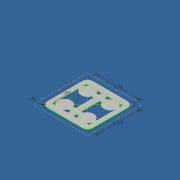
# Autodesk Inventor part: PCB Dome Array Tape
Saved by Autodesk Inventor 2016 (Build 200138000, 138)
## iProperties
Created: 2016-02-25
Part Number: PCB Dome Array Tape
Material: Generic
Document SubType Name: Modeling
Designer: Sam Clay
Density: 1 g/cm^3
Appearance: Default
Author: Sam Clay
Autodesk Inventor part; units mm, degrees
ref_plane "YZ Plane" through (0, 0, 0) normal (1, 0, 0) x (0, 1, 0)
ref_plane "XZ Plane" through (0, 0, 0) normal (0, 1, 0) x (-1, 0, 0)
ref_plane "XY Plane" through (0, 0, 0) normal (0, 0, 1) x (1, 0, 0)
sketch "Sketch1" plane through (0, 0, 0) normal (0, 1, 0) x (-1, 0, 0)
  line L0 (-15.24, 11.7348) -> (-15.24, -11.7348)
  line L1 (-11.7348, -15.24) -> (11.7348, -15.24)
  line L2 (15.24, -11.7348) -> (15.24, 11.7348)
  line L3 (11.7348, 15.24) -> (-11.7348, 15.24)
  line L4 (-15.24, 15.24) -> (15.24, -15.24) construction
  line L5 (-15.24, -15.24) -> (15.24, 15.24) construction
  arc A0 (15.24, 11.7348) -> (11.7348, 15.24) centre (11.7348, 11.7348) ccw
  arc A1 (11.7348, -15.24) -> (15.24, -11.7348) centre (11.7348, -11.7348) ccw
  arc A2 (-15.24, -11.7348) -> (-11.7348, -15.24) centre (-11.7348, -11.7348) ccw
  arc A3 (-11.7348, 15.24) -> (-15.24, 11.7348) centre (-11.7348, 11.7348) ccw
  line L6 (-18.4479, 18.3502) -> (18.4026, 18.3502) construction
  line L7 (18.4026, 18.3502) -> (18.4026, -18.5003) construction
  line L8 (18.4026, -18.5003) -> (-18.4479, -18.5003) construction
  line L9 (-18.4479, -18.5003) -> (-18.4479, 18.3502) construction
  line L10 (12.7, 11.7348) -> (12.7, 9.1616)
  arc A4 (11.7348, -12.7) -> (12.7, -11.7348) centre (11.7348, -11.7348) ccw
  line L11 (11.7348, -12.7) -> (-11.7348, -12.7)
  arc A5 (-12.7, -11.7348) -> (-11.7348, -12.7) centre (-11.7348, -11.7348) ccw
  line L12 (-12.7, -11.7348) -> (-12.7, -9.2677)
  arc A6 (-11.7348, 12.7) -> (-12.7, 11.7348) centre (-11.7348, 11.7348) ccw
  line L13 (-11.7348, 12.7) -> (11.7348, 12.7)
  arc A7 (12.7, 11.7348) -> (11.7348, 12.7) centre (11.7348, 11.7348) ccw
  line L14 (12.7, 9.1616) -> (1.5905, 9.1616)
  line L15 (-12.7, 9.1616) -> (-12.7, 11.7348)
  line L16 (-12.7, 11.7348) -> (-1.7389, 11.7348)
  line L17 (12.7, 11.7348) -> (12.7, 9.1616)
  line L18 (12.7, -9.2677) -> (1.5905, -9.2677)
  line L19 (-12.7, -9.2677) -> (-12.7, -11.7348)
  line L20 (-12.7, -11.7348) -> (-1.7389, -11.7348)
  line L21 (12.7, -11.7348) -> (12.7, -9.2677)
  line L22 (-12.7, 9.1616) -> (-12.7, 11.7348)
  line L23 (12.7, 6.4035) -> (6.4035, 6.4035)
  line L24 (-12.7, 6.4035) -> (-12.7, -6.3499)
  line L25 (-12.7, -6.3499) -> (-1.7389, -6.3499)
  line L26 (12.7, -6.3499) -> (12.7, 6.4035)
  line L27 (12.7, -6.3499) -> (12.7, -9.2677)
  line L28 (12.7, 6.4035) -> (12.7, -6.3499)
  line L29 (12.7, 9.1616) -> (12.7, 6.4035)
  line L30 (12.7, -9.2677) -> (12.7, -11.7348)
  line L31 (-12.7, -9.2677) -> (-12.7, -6.3499)
  line L32 (-12.7, -6.3499) -> (-12.7, 6.4035)
  line L33 (-12.7, 6.4035) -> (-12.7, 9.1616)
  line L34 (1.5905, 11.7348) -> (-1.7389, 11.7348)
  line L35 (-1.7389, 11.7348) -> (-1.7389, -11.7348)
  line L36 (-1.7389, -11.7348) -> (1.5905, -11.7348)
  line L37 (1.5905, -11.7348) -> (1.5905, 11.7348)
  line L38 (1.5905, 11.7348) -> (12.7, 11.7348)
  line L39 (-1.7389, 11.7348) -> (1.5905, 11.7348)
  line L40 (1.5905, -11.7348) -> (12.7, -11.7348)
  line L41 (-1.7389, -11.7348) -> (1.5905, -11.7348)
  line L42 (1.5905, 9.1616) -> (-1.7389, 9.1616)
  line L43 (-1.7389, 9.1616) -> (-12.7, 9.1616)
  line L44 (6.4035, 6.4035) -> (1.5905, 6.4035)
  line L45 (1.5905, 6.4035) -> (-1.7389, 6.4035)
  line L46 (6.3499, -6.3499) -> (12.7, -6.3499)
  line L47 (1.5905, -6.3499) -> (6.3499, -6.3499)
  line L48 (1.5905, -9.2677) -> (-1.7389, -9.2677)
  line L49 (-1.7389, -9.2677) -> (-12.7, -9.2677)
  line L50 (-1.7389, -6.3499) -> (1.5905, -6.3499)
  line L51 (-1.7389, 6.4035) -> (-12.7, 6.4035)
  point P0 (0, 0)
  dimension "d15" = 30.48
  dimension "d16" = 30.48
  dimension "d17" = 3.5052
  dimension "d21" = 2.54
  constraints: 96 end point, 67 parallel, 21 point on line, 17 perpendicular, 16 point on circle, 11 horizontal, 8 centre point, 8 tangent, 3 equal radius, 2 midpoint, 1 vertical, 6 other
  measures "d15" distance of L4.start L5.start
  measures "d16" distance of L4.end L5.start
  measures "d17" radius of A0
  measures "d21" distance between parallel lines of L2 L10
extrude "Extrusion1" add sketch "Sketch1" along normal blind 0.2286 contours A3 L3 A0 L2 A1 L1 A2 L0 | L38 L34 L16 A6 L13 A7 | L29 L23 L44 L37 L14 | L37 L42 L35 L34 | L37 L45 L35 L42 | L37 L50 L35 L45 | L35 L51 L33 L43 | L27 L18 L37 L47 L46 | L37 L48 L35 L50 | L37 L36 L35 L48 | L35 L49 L31 L25 | A4 L11 A5 L20 L36 L40
sketch "Sketch2" plane through (0, 0, 0) normal (0, 1, 0) x (-1, 0, 0)
  circle A0 centre (7.8475, 7.62) radius 4.445
  line L0 (17.2095, 0) -> (-17.2095, 0) projected
  line L1 (0, -17.2095) -> (0, 17.2095) projected
  circle A1 centre (-7.62, 7.8475) radius 4.445
  circle A2 centre (-7.8475, -7.62) radius 4.445
  circle A3 centre (7.62, -7.8475) radius 4.445
  point P0 (0, 0)
  dimension "d24" = 8.89
  dimension "d25" = 7.62
  dimension "d28" = 360
  constraints: 4 centre point, 9 other
  measures "d24" diameter of A0
  measures "d25" vertical distance of point (0, 0) A0.centre
extrude "Extrusion2" add sketch "Sketch2" along normal blind 0.3302 draft -86 separate body
body "Solid1"
body "Solid2"
